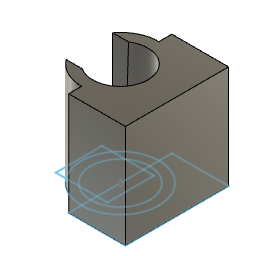
L-shape Nozzle Fitting Connector Prototype (Autodesk Fusion 360 design; units mm, degrees)
Autodesk Fusion 360 part; units mm, degrees
note: some values were not read from the file. Set by a fixed rule: which sketch regions a step uses.
sketch "Sketch1" plane through (0, 0, 0) normal (0, 0, 1) x (1, 0, 0)
  line L0 (-25, 10) -> (-14, 10)
  line L1 (-14, 10) -> (-14, -10)
  line L2 (-14, -10) -> (-25, -10)
  line L3 (-25, -10) -> (-25, 10)
  circle A0 centre (-25, 0) radius 7.5
  circle A1 centre (-25, 0) radius 5.7
  line L4 (-33, 4.5) -> (-23, 4.5)
  line L5 (-23, 4.5) -> (-23, -4.5)
  line L6 (-23, -4.5) -> (-33, -4.5)
  line L7 (-33, -4.5) -> (-33, 4.5)
  dimension "d1" = 11
  dimension "d2" = 20
  dimension "d3" = 15
  dimension "d6" = 11.4
  dimension "d9" = 9
  dimension "d10" = 10
  constraint horizontal L0
  constraint vertical L1
  constraint horizontal L2
  constraint vertical L3
  constraint midpoint L3 A0.centre
  constraint concentric A0 A1
  constraint horizontal L4
  constraint vertical L5
  constraint horizontal L6
  constraint vertical L7
  measures "d1" distance of L0.start L0.end
  measures "d2" distance of L0.start L2.end
  measures "d3" diameter of A0
  measures "d6" diameter of A1
  measures "d9" distance of L4.start L6.end
  measures "d10" distance of L4.start L4.end
extrude "Extrude1" add sketch "Sketch1" along normal blind 20 contours L0 L1 L2 L3 A0 | L3 A0 A1 | L3 A0 A1 L4 | L3 A1 L4 L5 L6 | L3 A1 L4 | A0 A1 L4 L6 | L3 L4 L5 L6 | L3 A1 L4 L6 | L3 A0 A1 L6 | L3 A1 L6
extrude "Extrude2" cut sketch "Sketch1" along normal blind 20 draft -1 contours L3 A1 L4 L5 L6 | L3 A1 L4 | L3 L4 L5 L6 | L3 A1 L4 L6 | L3 A1 L6
extrude "Extrude3" cut sketch "Sketch1" along normal blind 20 contours A0 A1 L4 L6 | A0 L4 L6 L7 | L3 A1 L4 L6
